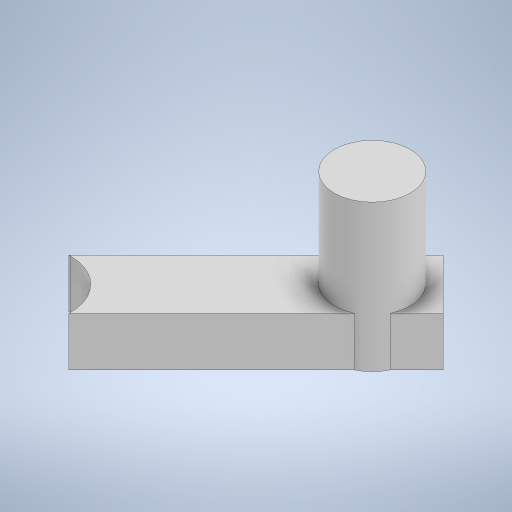
# Autodesk Inventor part: hjørner holder
Saved by Autodesk Inventor 2024 (Build 280153000, 153)
## iProperties
Created: 2024-03-27
Part Number: hjørner holder
Material: Generic
Document SubType Name: Modeling
Designer: laura
Density: 1 g/cm^3
Appearance: Default
Author: laura
Autodesk Inventor part; units mm, degrees
ref_plane "YZ Plane" through (0, 0, 0) normal (1, 0, 0) x (0, 1, 0)
ref_plane "XZ Plane" through (0, 0, 0) normal (0, 1, 0) x (-1, 0, 0)
ref_plane "XY Plane" through (0, 0, 0) normal (0, 0, 1) x (1, 0, 0)
sketch "Sketch1" plane through (0, 0, 0) normal (0, 1, 0) x (-1, 0, 0)
  circle A0 centre (0.0391, 0.0653) radius 7.75
  line L0 (25.8724, 25.8987) -> (36.2057, 25.8987)
  line L1 (25.8724, 36.232) -> (25.8724, 25.8987)
  line L2 (36.2057, 25.8987) -> (-2.0324, -12.3395)
  line L3 (25.8724, 36.232) -> (-12.3657, -2.0061)
  line L4 (25.8724, 36.232) -> (79.9493, 36.232) construction
  line L5 (-12.3657, -2.0061) -> (-2.0324, -12.3395)
  point P0 (0, 0)
  point P1 (-53.1731, 12.2093)
  point P2 (3.379, -6.928)
  point P3 (-6.9543, 3.4053)
  point P4 (-3.3009, 7.0587)
  point P5 (7.0324, -3.2747)
  dimension "d0" = 15.5
  dimension "d1" = 135
  constraints: 12 end point, 2 horizontal, 1 centre point, 1 equal length, 1 perpendicular
  measures "d0" diameter of A0
  measures "d1" angle of L3 L4
extrude "Extrusion1" add sketch "Sketch1" along normal blind 10 contours A0 L3 L1 L0 L2 | A0 L2 L5 L3
extrude "Extrusion2" add sketch "Sketch1" along normal blind 30 contours A0 L2 L3 | L3 A0 | A0 L2
fillet "Fillet1" radius 10 1 edges at (-25.8724, 5, 25.8987)
body "Solid1"
